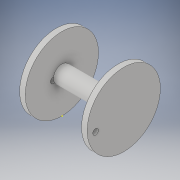
# Autodesk Inventor part: SpoolNoCenterHole1
Saved by Autodesk Inventor 2019 (Build 230136000, 136)
## iProperties
Created: 2019-01-13
Part Number: SpoolNoCenterHole1
Material: Generic
Document SubType Name: Modeling
Designer: Kepler
Density: 1 g/cm^3
Appearance: Default
Author: Kepler
Autodesk Inventor part; units mm, degrees
ref_plane "YZ Plane" through (0, 0, 0) normal (1, 0, 0) x (0, 1, 0)
ref_plane "XZ Plane" through (0, 0, 0) normal (0, 1, 0) x (-1, 0, 0)
ref_plane "XY Plane" through (0, 0, 0) normal (0, 0, 1) x (1, 0, 0)
sketch "Sketch1" plane through (0, 0, 0) normal (0, 0, 1) x (1, 0, 0)
  line L0 (0, 0) -> (0, 13)
  line L1 (0, 13) -> (24, 13)
  line L2 (24, 13) -> (24, 0)
  line L3 (24, 0) -> (22, 0)
  line L4 (22, 0) -> (22, 10)
  line L5 (22, 10) -> (2, 10)
  line L6 (2, 10) -> (2, 0)
  line L7 (2, 0) -> (0, 0)
  dimension "d0" = 13
  dimension "d1" = 24
  dimension "d2" = 2
  dimension "d3" = 10
  dimension "d4" = 20
  constraints: 16 end point, 6 perpendicular, 2 parallel, 1 vertical
  measures "d0" distance of L0.start L0.end
  measures "d1" distance of L0.end L1.end
  measures "d2" distance of L2.end L3.end
  measures "d3" distance of L3.end L4.end
  measures "d4" distance of L4.end L5.end
revolve "Revolution1" add sketch "Sketch1" angle 360 about axis through (0, 13, 0) along (1, 0, 0)
sketch "Sketch2" plane through (2, 13, 0) normal (1, 0, 0) x (0, 0, -1)
  point P0 (0, -13)
  point P1 (-3.0767, -0.4716)
hole "Hole1" at (2, 12.5284, 3.0767) direction (-1, 0, 0) diameter 2 end through all
sketch "Sketch3" plane through (24, 13, 0) normal (1, 0, 0) x (0, 0, -1)
  point P0 (0, -13)
  point P1 (-10.0295, -1.8525)
hole "Hole2" at (24, 11.1475, 10.0295) direction (-1, 0, 0) diameter 2 depth 8 tip angle 118
sketch "Sketch4" plane through (2, 13, 0) normal (1, 0, 0) x (0, 0, -1)
  point P0 (0, -13)
sketch "Sketch5" plane through (2, 13, 0) normal (1, 0, 0) x (0, 0, -1)
  point P0 (0, -13)
body "Solid1"
